Autodesk Inventor part; units mm, degrees
(part 3 of 3)
sketch "Sketch5" plane through (203.2, 0, 0) normal (0, 0, -1) x (-1, 0, 0)
  line L0 (0, 0) -> (203.2, 0) projected
  line L1 (0, 0) -> (0, -25.4) projected
  line L2 (203.2, -25.4) -> (0, -25.4) projected
  line L3 (203.2, 0) -> (203.2, -25.4) projected
  line L4 (50.8, -8.636) -> (152.4, -8.636) construction
  line L5 (152.4, -8.636) -> (152.4, -16.764) construction
  line L6 (152.4, -16.764) -> (50.8, -16.764) construction
  line L7 (50.8, -16.764) -> (50.8, -8.636) construction
  line L8 (60.5212, -15.7381) -> (62.5762, -9.6421)
  line L9 (62.5762, -9.6421) -> (63.5741, -9.6421)
  line L10 (63.5741, -9.6421) -> (65.6292, -15.7381)
  line L11 (65.6292, -15.7381) -> (64.7745, -15.7381)
  line L12 (64.7745, -15.7381) -> (64.2212, -14.0338)
  line L13 (64.2212, -14.0338) -> (61.8945, -14.0338)
  line L14 (61.8945, -14.0338) -> (61.3412, -15.7381)
  line L15 (61.3412, -15.7381) -> (60.5212, -15.7381)
  line L16 (63.9989, -13.3422) -> (63.0554, -10.472)
  line L17 (63.0554, -10.472) -> (62.1168, -13.3422)
  line L18 (62.1168, -13.3422) -> (63.9989, -13.3422)
  line L19 (70.6285, -9.6421) -> (68.529, -15.7381)
  line L20 (68.529, -15.7381) -> (67.6546, -15.7381)
  line L21 (67.6546, -15.7381) -> (65.5551, -9.6421)
  line L22 (65.5551, -9.6421) -> (66.4245, -9.6421)
  line L23 (66.4245, -9.6421) -> (68.114, -14.7057)
  line L24 (68.114, -14.7057) -> (69.8035, -9.6421)
  line L25 (69.8035, -9.6421) -> (70.6285, -9.6421)
  line L26 (71.2114, -15.7381) -> (71.2114, -9.6421)
  line L27 (71.2114, -9.6421) -> (75.0251, -9.6421)
  line L28 (75.0251, -9.6421) -> (75.0251, -10.3634)
  line L29 (75.0251, -10.3634) -> (72.0216, -10.3634)
  line L30 (72.0216, -10.3634) -> (72.0216, -12.0331)
  line L31 (72.0216, -12.0331) -> (74.8226, -12.0331)
  line L32 (74.8226, -12.0331) -> (74.8226, -12.7543)
  line L33 (74.8226, -12.7543) -> (72.0216, -12.7543)
  line L34 (72.0216, -12.7543) -> (72.0216, -15.0169)
  line L35 (72.0216, -15.0169) -> (75.0251, -15.0169)
  line L36 (75.0251, -15.0169) -> (75.0251, -15.7381)
  line L37 (75.0251, -15.7381) -> (71.2114, -15.7381)
  line L38 (80.632, -15.7381) -> (79.5798, -15.7381)
  line L39 (79.5798, -15.7381) -> (77.6532, -13.3126)
  line L40 (77.6532, -13.3126) -> (76.7245, -13.3126)
  line L41 (76.7245, -13.3126) -> (76.7245, -15.7381)
  line L42 (76.7245, -15.7381) -> (75.9143, -15.7381)
  line L43 (75.9143, -15.7381) -> (75.9143, -9.6421)
  line L44 (75.9143, -9.6421) -> (77.4852, -9.6421)
  spline S0 degree 2 poles (77.4852, -9.6421) (78.0089, -9.6421) (78.7153, -9.7557) (79.0364, -9.9632) knots 0 0 0 1 2 2 2
  spline S1 degree 2 poles (79.0364, -9.9632) (79.3575, -10.1707) (79.728, -10.8178) (79.728, -11.297) knots 0 0 0 1 2 2 2
  spline S2 degree 2 poles (79.728, -11.297) (79.728, -11.9639) (79.0463, -12.868) (78.4634, -13.0853) knots 0 0 0 1 2 2 2
  line L45 (78.4634, -13.0853) -> (80.632, -15.7381)
  spline S3 degree 2 poles (78.8833, -11.3613) (78.8833, -11.0945) (78.6955, -10.6845) (78.4979, -10.5511) knots 0 0 0 1 2 2 2
  spline S4 degree 2 poles (78.4979, -10.5511) (78.325, -10.4375) (77.8656, -10.3436) (77.5297, -10.3436) knots 0 0 0 1 2 2 2
  line L46 (77.5297, -10.3436) -> (76.7245, -10.3436)
  line L47 (76.7245, -10.3436) -> (76.7245, -12.6358)
  line L48 (76.7245, -12.6358) -> (77.4358, -12.6358)
  spline S5 degree 2 poles (77.4358, -12.6358) (77.7866, -12.6358) (78.3448, -12.5123) (78.5375, -12.3196) knots 0 0 0 1 2 2 2
  spline S6 degree 2 poles (78.5375, -12.3196) (78.7153, -12.1517) (78.8833, -11.6774) (78.8833, -11.3613) knots 0 0 0 1 2 2 2
  line L49 (80.4591, -15.7381) -> (82.5142, -9.6421)
  line L50 (82.5142, -9.6421) -> (83.5121, -9.6421)
  line L51 (83.5121, -9.6421) -> (85.5671, -15.7381)
  line L52 (85.5671, -15.7381) -> (84.7125, -15.7381)
  line L53 (84.7125, -15.7381) -> (84.1592, -14.0338)
  line L54 (84.1592, -14.0338) -> (81.8325, -14.0338)
  line L55 (81.8325, -14.0338) -> (81.2792, -15.7381)
  line L56 (81.2792, -15.7381) -> (80.4591, -15.7381)
  line L57 (83.9369, -13.3422) -> (82.9934, -10.472)
  line L58 (82.9934, -10.472) -> (82.0548, -13.3422)
  line L59 (82.0548, -13.3422) -> (83.9369, -13.3422)
  spline S7 degree 2 poles (88.6991, -15.8567) (88.052, -15.8567) (86.98, -15.4615) (86.5947, -15.0613) knots 0 0 0 1 2 2 2
  spline S8 degree 2 poles (86.5947, -15.0613) (86.2093, -14.6563) (85.7993, -13.4608) (85.7993, -12.6852) knots 0 0 0 1 2 2 2
  spline S9 degree 2 poles (85.7993, -12.6852) (85.7993, -11.9491) (86.2143, -10.7833) (86.5996, -10.3683) knots 0 0 0 1 2 2 2
  spline S10 degree 2 poles (86.5996, -10.3683) (86.9701, -9.9682) (88.0569, -9.5334) (88.704, -9.5334) knots 0 0 0 1 2 2 2
  spline S11 degree 2 poles (88.704, -9.5334) (89.0153, -9.5334) (89.5784, -9.6224) (89.8353, -9.7014) knots 0 0 0 1 2 2 2
  spline S12 degree 2 poles (89.8353, -9.7014) (90.0428, -9.7607) (90.5467, -9.978) (90.6998, -10.0571) knots 0 0 0 1 2 2 2
  line L60 (90.6998, -10.0571) -> (90.6998, -11.0352)
  line L61 (90.6998, -11.0352) -> (90.6307, -11.0352)
  spline S13 degree 2 poles (90.6307, -11.0352) (90.4775, -10.9018) (90.1564, -10.6598) (89.86, -10.5214) knots 0 0 0 1 2 2 2
  spline S14 degree 2 poles (89.86, -10.5214) (89.613, -10.3979) (88.9757, -10.2349) (88.6102, -10.2349) knots 0 0 0 1 2 2 2
  spline S15 degree 2 poles (88.6102, -10.2349) (87.7309, -10.2349) (86.6441, -11.5589) (86.6441, -12.6605) knots 0 0 0 1 2 2 2
  spline S16 degree 2 poles (86.6441, -12.6605) (86.6441, -13.273) (86.9306, -14.1919) (87.2023, -14.5081) knots 0 0 0 1 2 2 2
  spline S17 degree 2 poles (87.2023, -14.5081) (87.4641, -14.8242) (88.2051, -15.1552) (88.6695, -15.1552) knots 0 0 0 1 2 2 2
  spline S18 degree 2 poles (88.6695, -15.1552) (89.0103, -15.1552) (89.6921, -15.0564) (89.9242, -14.9576) knots 0 0 0 1 2 2 2
  line L62 (89.9242, -14.9576) -> (89.9242, -13.3817)
  line L63 (89.9242, -13.3817) -> (88.5114, -13.3817)
  line L64 (88.5114, -13.3817) -> (88.5114, -12.6704)
  line L65 (88.5114, -12.6704) -> (90.7245, -12.6704)
  line L66 (90.7245, -12.6704) -> (90.7245, -15.333)
  spline S19 degree 2 poles (90.7245, -15.333) (90.5714, -15.4022) (90.0477, -15.6146) (89.8254, -15.6788) knots 0 0 0 1 2 2 2
  spline S20 degree 2 poles (89.8254, -15.6788) (89.5241, -15.7678) (89.04, -15.8567) (88.6991, -15.8567) knots 0 0 0 1 2 2 2
  line L67 (91.7422, -15.7381) -> (91.7422, -9.6421)
  line L68 (91.7422, -9.6421) -> (95.5559, -9.6421)
  line L69 (95.5559, -9.6421) -> (95.5559, -10.3634)
  line L70 (95.5559, -10.3634) -> (92.5523, -10.3634)
  line L71 (92.5523, -10.3634) -> (92.5523, -12.0331)
  line L72 (92.5523, -12.0331) -> (95.3533, -12.0331)
  line L73 (95.3533, -12.0331) -> (95.3533, -12.7543)
  line L74 (95.3533, -12.7543) -> (92.5523, -12.7543)
  line L75 (92.5523, -12.7543) -> (92.5523, -15.0169)
  line L76 (92.5523, -15.0169) -> (95.5559, -15.0169)
  line L77 (95.5559, -15.0169) -> (95.5559, -15.7381)
  line L78 (95.5559, -15.7381) -> (91.7422, -15.7381)
  line L79 (98.4063, -15.7381) -> (100.4613, -9.6421)
  line L80 (100.4613, -9.6421) -> (101.4592, -9.6421)
  line L81 (101.4592, -9.6421) -> (103.5143, -15.7381)
  line L82 (103.5143, -15.7381) -> (102.6596, -15.7381)
  line L83 (102.6596, -15.7381) -> (102.1064, -14.0338)
  line L84 (102.1064, -14.0338) -> (99.7796, -14.0338)
  line L85 (99.7796, -14.0338) -> (99.2263, -15.7381)
  line L86 (99.2263, -15.7381) -> (98.4063, -15.7381)
  line L87 (101.8841, -13.3422) -> (100.9405, -10.472)
  line L88 (100.9405, -10.472) -> (100.0019, -13.3422)
  line L89 (100.0019, -13.3422) -> (101.8841, -13.3422)
  line L90 (109.3188, -15.7381) -> (108.5086, -15.7381)
  line L91 (108.5086, -15.7381) -> (108.5086, -10.4869)
  line L92 (108.5086, -10.4869) -> (106.9179, -14.0585)
  line L93 (106.9179, -14.0585) -> (106.4239, -14.0585)
  line L94 (106.4239, -14.0585) -> (104.8481, -10.4869)
  line L95 (104.8481, -10.4869) -> (104.8481, -15.7381)
  line L96 (104.8481, -15.7381) -> (104.0922, -15.7381)
  line L97 (104.0922, -15.7381) -> (104.0922, -9.6421)
  line L98 (104.0922, -9.6421) -> (105.1988, -9.6421)
  line L99 (105.1988, -9.6421) -> (106.7203, -13.0359)
  line L100 (106.7203, -13.0359) -> (108.1925, -9.6421)
  line L101 (108.1925, -9.6421) -> (109.3188, -9.6421)
  line L102 (109.3188, -9.6421) -> (109.3188, -15.7381)
  spline S21 degree 2 poles (114.407, -11.4798) (114.407, -11.875) (114.1255, -12.5864) (113.8735, -12.8334) knots 0 0 0 1 2 2 2
  spline S22 degree 2 poles (113.8735, -12.8334) (113.5573, -13.1446) (112.7027, -13.4657) (112.0506, -13.4657) knots 0 0 0 1 2 2 2
  line L103 (112.0506, -13.4657) -> (111.364, -13.4657)
  line L104 (111.364, -13.4657) -> (111.364, -15.7381)
  line L105 (111.364, -15.7381) -> (110.5538, -15.7381)
  line L106 (110.5538, -15.7381) -> (110.5538, -9.6421)
  line L107 (110.5538, -9.6421) -> (112.0852, -9.6421)
  spline S23 degree 2 poles (112.0852, -9.6421) (112.6286, -9.6421) (113.3894, -9.82) (113.6808, -10.0225) knots 0 0 0 1 2 2 2
  spline S24 degree 2 poles (113.6808, -10.0225) (114.0217, -10.2547) (114.407, -10.971) (114.407, -11.4798) knots 0 0 0 1 2 2 2
  spline S25 degree 2 poles (113.5623, -11.5045) (113.5623, -11.1884) (113.3449, -10.724) (113.1226, -10.5758) knots 0 0 0 1 2 2 2
  spline S26 degree 2 poles (113.1226, -10.5758) (112.93, -10.4473) (112.4162, -10.3436) (112.0358, -10.3436) knots 0 0 0 1 2 2 2
  line L108 (112.0358, -10.3436) -> (111.364, -10.3436)
  line L109 (111.364, -10.3436) -> (111.364, -12.7741)
  line L110 (111.364, -12.7741) -> (111.9173, -12.7741)
  spline S27 degree 2 poles (111.9173, -12.7741) (112.4113, -12.7741) (113.0189, -12.616) (113.2165, -12.4085) knots 0 0 0 1 2 2 2
  spline S28 degree 2 poles (113.2165, -12.4085) (113.3993, -12.2258) (113.5623, -11.796) (113.5623, -11.5045) knots 0 0 0 1 2 2 2
  line L111 (118.7098, -15.7381) -> (115.1777, -15.7381)
  line L112 (115.1777, -15.7381) -> (115.1777, -9.6421)
  line L113 (115.1777, -9.6421) -> (115.9878, -9.6421)
  line L114 (115.9878, -9.6421) -> (115.9878, -15.0169)
  line L115 (115.9878, -15.0169) -> (118.7098, -15.0169)
  line L116 (118.7098, -15.0169) -> (118.7098, -15.7381)
  line L117 (121.4713, -15.7381) -> (119.1099, -15.7381)
  line L118 (119.1099, -15.7381) -> (119.1099, -15.1157)
  line L119 (119.1099, -15.1157) -> (119.8855, -15.1157)
  line L120 (119.8855, -15.1157) -> (119.8855, -10.2646)
  line L121 (119.8855, -10.2646) -> (119.1099, -10.2646)
  line L122 (119.1099, -10.2646) -> (119.1099, -9.6421)
  line L123 (119.1099, -9.6421) -> (121.4713, -9.6421)
  line L124 (121.4713, -9.6421) -> (121.4713, -10.2646)
  line L125 (121.4713, -10.2646) -> (120.6957, -10.2646)
  line L126 (120.6957, -10.2646) -> (120.6957, -15.1157)
  line L127 (120.6957, -15.1157) -> (121.4713, -15.1157)
  line L128 (121.4713, -15.1157) -> (121.4713, -15.7381)
  line L129 (123.8968, -15.7381) -> (123.8968, -10.3634)
  line L130 (123.8968, -10.3634) -> (121.8517, -10.3634)
  line L131 (121.8517, -10.3634) -> (121.8517, -9.6421)
  line L132 (121.8517, -9.6421) -> (126.7522, -9.6421)
  line L133 (126.7522, -9.6421) -> (126.7522, -10.3634)
  line L134 (126.7522, -10.3634) -> (124.707, -10.3634)
  line L135 (124.707, -10.3634) -> (124.707, -15.7381)
  line L136 (124.707, -15.7381) -> (123.8968, -15.7381)
  spline S29 degree 2 poles (129.4988, -15.8666) (128.9604, -15.8666) (128.1601, -15.585) (127.8785, -15.3034) knots 0 0 0 1 2 2 2
  spline S30 degree 2 poles (127.8785, -15.3034) (127.5574, -14.9872) (127.2956, -14.098) (127.2956, -13.4459) knots 0 0 0 1 2 2 2
  line L137 (127.2956, -13.4459) -> (127.2956, -9.6421)
  line L138 (127.2956, -9.6421) -> (128.1057, -9.6421)
  line L139 (128.1057, -9.6421) -> (128.1057, -13.4459)
  spline S31 degree 2 poles (128.1057, -13.4459) (128.1057, -13.8708) (128.2144, -14.4438) (128.3676, -14.676) knots 0 0 0 1 2 2 2
  spline S32 degree 2 poles (128.3676, -14.676) (128.5306, -14.923) (129.0937, -15.175) (129.4988, -15.175) knots 0 0 0 1 2 2 2
  spline S33 degree 2 poles (129.4988, -15.175) (129.8792, -15.175) (130.472, -14.923) (130.635, -14.676) knots 0 0 0 1 2 2 2
  spline S34 degree 2 poles (130.635, -14.676) (130.7882, -14.4438) (130.8969, -13.8757) (130.8969, -13.4657) knots 0 0 0 1 2 2 2
  line L140 (130.8969, -13.4657) -> (130.8969, -9.6421)
  line L141 (130.8969, -9.6421) -> (131.707, -9.6421)
  line L142 (131.707, -9.6421) -> (131.707, -13.4459)
  spline S35 degree 2 poles (131.707, -13.4459) (131.707, -14.0832) (131.4501, -14.9922) (131.1241, -15.3034) knots 0 0 0 1 2 2 2
  spline S36 degree 2 poles (131.1241, -15.3034) (130.8326, -15.5899) (130.062, -15.8666) (129.4988, -15.8666) knots 0 0 0 1 2 2 2
  spline S37 degree 2 poles (137.6746, -12.6951) (137.6746, -13.5299) (136.9978, -14.8736) (136.4297, -15.2491) knots 0 0 0 1 2 2 2
  spline S38 degree 2 poles (136.4297, -15.2491) (135.9653, -15.5405) (135.0119, -15.7381) (134.2709, -15.7381) knots 0 0 0 1 2 2 2
  line L143 (134.2709, -15.7381) -> (132.8679, -15.7381)
  line L144 (132.8679, -15.7381) -> (132.8679, -9.6421)
  line L145 (132.8679, -9.6421) -> (134.2561, -9.6421)
  spline S39 degree 2 poles (134.2561, -9.6421) (135.1156, -9.6421) (136.0938, -9.899) (136.4396, -10.1262) knots 0 0 0 1 2 2 2
  spline S40 degree 2 poles (136.4396, -10.1262) (137.0274, -10.5165) (137.6746, -11.8059) (137.6746, -12.6951) knots 0 0 0 1 2 2 2
  spline S41 degree 2 poles (136.8298, -12.6852) (136.8298, -11.9837) (136.3655, -10.9907) (135.9061, -10.7092) knots 0 0 0 1 2 2 2
  spline S42 degree 2 poles (135.9061, -10.7092) (135.58, -10.5165) (134.8439, -10.3436) (134.2956, -10.3436) knots 0 0 0 1 2 2 2
  line L146 (134.2956, -10.3436) -> (133.6781, -10.3436)
  line L147 (133.6781, -10.3436) -> (133.6781, -15.0366)
  line L148 (133.6781, -15.0366) -> (134.2956, -15.0366)
  spline S43 degree 2 poles (134.2956, -15.0366) (134.8341, -15.0366) (135.6492, -14.8637) (135.9802, -14.6316) knots 0 0 0 1 2 2 2
  spline S44 degree 2 poles (135.9802, -14.6316) (136.405, -14.345) (136.8298, -13.3965) (136.8298, -12.6852) knots 0 0 0 1 2 2 2
  line L149 (138.5539, -15.7381) -> (138.5539, -9.6421)
  line L150 (138.5539, -9.6421) -> (142.3676, -9.6421)
  line L151 (142.3676, -9.6421) -> (142.3676, -10.3634)
  line L152 (142.3676, -10.3634) -> (139.3641, -10.3634)
  line L153 (139.3641, -10.3634) -> (139.3641, -12.0331)
  line L154 (139.3641, -12.0331) -> (142.1651, -12.0331)
  line L155 (142.1651, -12.0331) -> (142.1651, -12.7543)
  line L156 (142.1651, -12.7543) -> (139.3641, -12.7543)
  line L157 (139.3641, -12.7543) -> (139.3641, -15.0169)
  line L158 (139.3641, -15.0169) -> (142.3676, -15.0169)
  line L159 (142.3676, -15.0169) -> (142.3676, -15.7381)
  line L160 (142.3676, -15.7381) -> (138.5539, -15.7381)
  dimension "d26" = 203.2
  dimension "d27" = 25.4
  dimension "d28" = 101.6
  dimension "d29" = 8.128
  dimension "d30" = 8.636
  dimension "d31" = 50.8
  constraints: 2 other
  measures "d26" distance of L0.start L0.end
  measures "d27" distance of L0.start L1.end
  measures "d28" distance of L4.start L4.end
  measures "d29" distance of L6.end L4.start
  measures "d30" distance between parallel lines of L0 L4
  measures "d31" distance between parallel lines of L1 L7
extrude "Extrusion5" cut sketch "Sketch5" against normal blind 2.54 contours L8 L9 L10 L11 L12 L13 L14 L15 | L19 L20 L21 L22 L23 L24 L25 | L26 L27 L28 L29 L30 L31 L32 L33 L34 L35 L36 L37 | L38 L49 L45 | L45 L49 L50 L51 L52 L53 L54 L55 L56 | L38 L39 L40 L41 L42 L43 L44 S0 S1 S2 L45 L49 | S7 S8 S9 S10 S11 S12 L60 L61 S13 S14 S15 S16 S17 S18 L62 L63 L64 L65 L66 S19 S20 | L67 L68 L69 L70 L71 L72 L73 L74 L75 L76 L77 L78 | L79 L80 L81 L82 L83 L84 L85 L86 | L90 L91 L92 L93 L94 L95 L96 L97 L98 L99 L100 L101 L102 | S21 S22 L103 L104 L105 L106 L107 S23 S24 | L111 L112 L113 L114 L115 L116 | L117 L118 L119 L120 L121 L122 L123 L124 L125 L126 L127 L128 | L129 L130 L131 L132 L133 L134 L135 L136 | S29 S30 L137 L138 L139 S31 S32 S33 S34 L140 L141 L142 S35 S36 | S37 S38 L143 L144 L145 S39 S40 | L149 L150 L151 L152 L153 L154 L155 L156 L157 L158 L159 L160
equation "\"d2\" = 0.5 * d3 - 0.5 * d5"
equation "\"d7\" = 0.5 * d4 - 0.5 * d6"
equation "\"d14\" = 0.5 * d10 - 0.5 * d12"
equation "\"d15\" = 0.5 * d11 - 0.5 * d13"
equation "\"d22\" = 0.5 * d19 - 0.5 * d21"
equation "\"d23\" = 0.5 * d18 - 0.5 * d20"
equation "\"d30\" = 0.5 * d27 - 0.5 * d29"
equation "\"d31\" = 0.5 * d26 - 0.5 * d28"
body "Solid1"
